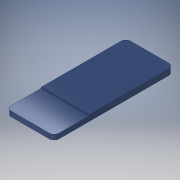
# Autodesk Inventor part: Adafruit-MicroLipoBatteryCharger
Saved by Autodesk Inventor 2019 (Build 230136000, 136)
## iProperties
Created: 2019-04-11
Part Number: Adafruit-MicroLipoBatteryCharger
Material: Generic
Document SubType Name: Modeling
Designer: Epsilon
Density: 1 g/cm^3
Appearance: Flaked Satin - Blue
Author: Epsilon
Autodesk Inventor part; units mm, degrees
ref_plane "YZ Plane" through (0, 0, 0) normal (1, 0, 0) x (0, 1, 0)
ref_plane "XZ Plane" through (0, 0, 0) normal (0, 1, 0) x (-1, 0, 0)
ref_plane "XY Plane" through (0, 0, 0) normal (0, 0, 1) x (1, 0, 0)
sketch "Sketch1" plane through (0, 0, 0) normal (0, 1, 0) x (-1, 0, 0)
  line L0 (1.27, 0) -> (10.922, 0)
  line L1 (12.192, -1.27) -> (12.192, -29.21)
  line L2 (10.922, -30.48) -> (1.27, -30.48)
  line L3 (0, -29.21) -> (0, -1.27)
  arc A0 (12.192, -1.27) -> (10.922, 0) centre (10.922, -1.27) ccw
  arc A1 (1.27, 0) -> (0, -1.27) centre (1.27, -1.27) ccw
  arc A2 (0, -29.21) -> (1.27, -30.48) centre (1.27, -29.21) ccw
  arc A3 (10.922, -30.48) -> (12.192, -29.21) centre (10.922, -29.21) ccw
  point P0 (0, 0)
  point P1 (12.192, -30.48)
  point P2 (12.192, 0)
  point P3 (0, -30.48)
  dimension "d0" = 12.192
  dimension "d1" = 30.48
  dimension "d2" = 1.27
  constraints: 8 end point, 8 point on circle, 8 point on line, 8 tangent, 4 centre point, 3 equal radius, 2 parallel, 1 horizontal, 1 perpendicular
  measures "d0" distance of point (12.192, -30.48) point (0, -30.48)
  measures "d1" distance of point (12.192, 0) point (12.192, -30.48)
  measures "d2" radius of A0
extrude "Extrusion1" add sketch "Sketch1" along normal blind 1.524
sketch "Sketch2" plane through (0, 1.524, 0) normal (0, 1, 0) x (1, 0, 0)
  line L0 (0, 1.27) -> (0, 29.21) projected
  line L1 (-12.192, 0) -> (0, 0)
  line L2 (0, 0) -> (0, 8.89)
  line L3 (0, 8.89) -> (-12.192, 8.89)
  line L4 (-12.192, 8.89) -> (-12.192, 0)
  arc A0 (-12.192, 1.27) -> (-10.922, 0) centre (-10.922, 1.27) ccw projected
  line L5 (-10.922, 0) -> (-1.27, 0) construction
  point P0 (0, 0)
  dimension "d5" = 8.89
  dimension "d6" = 12.192
  dimension "d7" = 9.652
  constraints: 10 end point, 2 horizontal, 2 parallel, 2 point on line, 1 perpendicular, 1 tangent
  measures "d5" distance of L2.end L1.end
  measures "d6" distance between parallel lines of L0 L4
  measures "d7" distance of L5.start L5.end
extrude "Extrusion2" cut sketch "Sketch2" against normal blind 0.254
body "Solid1"
